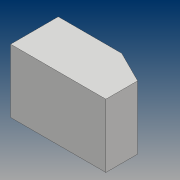
# Autodesk Inventor part: 42 (59000.000 mm^3)
Saved by Autodesk Inventor 2018 (Build 220112000, 112)
## iProperties
Created: 2020-09-18
Part Number: 42 (59000.000 mm^3)
Material: 一般
Document SubType Name: Modeling
Designer: 88697
Density: 1 g/cm^3
Appearance: 預設
Author: 88697
Autodesk Inventor part; units mm, degrees
ref_plane "YZ Plane" through (0, 0, 0) normal (1, 0, 0) x (0, 1, 0)
ref_plane "XZ Plane" through (0, 0, 0) normal (0, 1, 0) x (-1, 0, 0)
ref_plane "XY Plane" through (0, 0, 0) normal (0, 0, 1) x (1, 0, 0)
sketch "草圖1" plane through (0, 0, 0) normal (0, 0, 1) x (1, 0, 0)
  line L0 (0, 0) -> (60, 0)
  line L1 (60, 0) -> (60, 20)
  line L2 (60, 20) -> (0, 20)
  line L3 (0, 20) -> (0, 0)
  dimension "d0" = 60
  dimension "d1" = 20
  constraints: 8 end point, 2 parallel, 1 horizontal, 1 perpendicular
  measures "d0" distance of L0.start L0.end
  measures "d1" distance of L2.end L0.start
extrude "擠出1" add sketch "草圖1" along normal blind 40
sketch "草圖2" plane through (0, 0, 40) normal (0, 0, 1) x (1, 0, 0)
  line L0 (60, 20) -> (0, 20) projected
  line L1 (0, 20) -> (0, 30)
  line L2 (0, 30) -> (40, 30)
  line L3 (60, 0) -> (60, 20) projected
  line L4 (40, 30) -> (60, 20)
  line L5 (60, 20) -> (0, 20)
  point P0 (0, 0)
  dimension "d4" = 10
  dimension "d5" = 20
  constraints: 8 end point, 1 parallel, 1 perpendicular, 1 vertical
  measures "d4" distance of L0.end L1.end
  measures "d5" horizontal distance of L0.start L2.end
extrude "擠出2" add sketch "草圖2" against normal blind 10
sketch "草圖3" plane through (0, 0, 0) normal (0, 0, -1) x (-1, 0, 0)
  line L0 (0, 20) -> (-30, 20)
  line L1 (-30, 20) -> (-30, 40)
  line L2 (-30, 40) -> (0, 40)
  line L3 (0, 40) -> (0, 20)
  line L4 (-60, 20) -> (0, 20) projected
  line L5 (0, 20) -> (0, 0) projected
  dimension "d8" = 0
  dimension "d9" = 20
  dimension "d10" = 30
  dimension "d11" = 0
  constraints: 8 end point, 2 parallel, 1 horizontal, 1 perpendicular
  measures "d8" distance between parallel lines of L0 L4
  measures "d9" distance of L2.end L0.start
  measures "d10" distance of L1.end L2.end
  measures "d11" distance between parallel lines of L5 L3
extrude "擠出3" add sketch "草圖3" against normal blind 10
